Autodesk Inventor part; units mm, degrees
(part 12 of 15)
  arc A5313 (9.6668, 53.008) -> (9.5652, 53.008) centre (9.616, 53.008) ccw
  line L2483 (9.616, 52.992) -> (7.584, 52.992)
  arc A5314 (7.584, 53.0428) -> (7.584, 52.9412) centre (7.584, 52.992) ccw
  arc A5315 (9.616, 52.9412) -> (9.616, 53.0428) centre (9.616, 52.992) ccw
  line L2484 (7.584, 52.992) -> (7.584, 54.008)
  arc A5316 (7.6348, 54.008) -> (7.5332, 54.008) centre (7.584, 54.008) ccw
  arc A5317 (7.5332, 52.992) -> (7.6348, 52.992) centre (7.584, 52.992) ccw
  line L2485 (7.584, 54.008) -> (9.616, 54.008)
  arc A5318 (9.616, 53.9572) -> (9.616, 54.0588) centre (9.616, 54.008) ccw
  arc A5319 (7.584, 54.0588) -> (7.584, 53.9572) centre (7.584, 54.008) ccw
  line L2486 (9.616, 54.008) -> (9.616, 52.992)
  arc A5320 (9.5652, 52.992) -> (9.6668, 52.992) centre (9.616, 52.992) ccw
  arc A5321 (9.6668, 54.008) -> (9.5652, 54.008) centre (9.616, 54.008) ccw
  line L2487 (9.616, 53.992) -> (7.584, 53.992)
  arc A5322 (7.584, 54.0428) -> (7.584, 53.9412) centre (7.584, 53.992) ccw
  arc A5323 (9.616, 53.9412) -> (9.616, 54.0428) centre (9.616, 53.992) ccw
  line L2488 (7.584, 53.992) -> (7.584, 55.008)
  arc A5324 (7.6348, 55.008) -> (7.5332, 55.008) centre (7.584, 55.008) ccw
  arc A5325 (7.5332, 53.992) -> (7.6348, 53.992) centre (7.584, 53.992) ccw
  line L2489 (7.584, 55.008) -> (9.616, 55.008)
  arc A5326 (9.616, 54.9572) -> (9.616, 55.0588) centre (9.616, 55.008) ccw
  arc A5327 (7.584, 55.0588) -> (7.584, 54.9572) centre (7.584, 55.008) ccw
  line L2490 (9.616, 55.008) -> (9.616, 53.992)
  arc A5328 (9.5652, 53.992) -> (9.6668, 53.992) centre (9.616, 53.992) ccw
  arc A5329 (9.6668, 55.008) -> (9.5652, 55.008) centre (9.616, 55.008) ccw
  line L2491 (-9.484, 38.892) -> (-11.516, 38.892)
  arc A5330 (-11.516, 38.9428) -> (-11.516, 38.8412) centre (-11.516, 38.892) ccw
  arc A5331 (-9.484, 38.8412) -> (-9.484, 38.9428) centre (-9.484, 38.892) ccw
  line L2492 (-11.516, 38.892) -> (-11.516, 39.908)
  arc A5332 (-11.4652, 39.908) -> (-11.5668, 39.908) centre (-11.516, 39.908) ccw
  arc A5333 (-11.5668, 38.892) -> (-11.4652, 38.892) centre (-11.516, 38.892) ccw
  line L2493 (-11.516, 39.908) -> (-9.484, 39.908)
  arc A5334 (-9.484, 39.8572) -> (-9.484, 39.9588) centre (-9.484, 39.908) ccw
  arc A5335 (-11.516, 39.9588) -> (-11.516, 39.8572) centre (-11.516, 39.908) ccw
  line L2494 (-9.484, 39.908) -> (-9.484, 38.892)
  arc A5336 (-9.5348, 38.892) -> (-9.4332, 38.892) centre (-9.484, 38.892) ccw
  arc A5337 (-9.4332, 39.908) -> (-9.5348, 39.908) centre (-9.484, 39.908) ccw
  line L2495 (-9.484, 39.892) -> (-11.516, 39.892)
  arc A5338 (-11.516, 39.9428) -> (-11.516, 39.8412) centre (-11.516, 39.892) ccw
  arc A5339 (-9.484, 39.8412) -> (-9.484, 39.9428) centre (-9.484, 39.892) ccw
  line L2496 (-11.516, 39.892) -> (-11.516, 40.908)
  arc A5340 (-11.4652, 40.908) -> (-11.5668, 40.908) centre (-11.516, 40.908) ccw
  arc A5341 (-11.5668, 39.892) -> (-11.4652, 39.892) centre (-11.516, 39.892) ccw
  line L2497 (-11.516, 40.908) -> (-9.484, 40.908)
  arc A5342 (-9.484, 40.8572) -> (-9.484, 40.9588) centre (-9.484, 40.908) ccw
  arc A5343 (-11.516, 40.9588) -> (-11.516, 40.8572) centre (-11.516, 40.908) ccw
  line L2498 (-9.484, 40.908) -> (-9.484, 39.892)
  arc A5344 (-9.5348, 39.892) -> (-9.4332, 39.892) centre (-9.484, 39.892) ccw
  arc A5345 (-9.4332, 40.908) -> (-9.5348, 40.908) centre (-9.484, 40.908) ccw
  line L2499 (11.616, 49.992) -> (9.584, 49.992)
  arc A5346 (9.584, 50.0428) -> (9.584, 49.9412) centre (9.584, 49.992) ccw
  arc A5347 (11.616, 49.9412) -> (11.616, 50.0428) centre (11.616, 49.992) ccw
  line L2500 (9.584, 49.992) -> (9.584, 51.008)
  arc A5348 (9.6348, 51.008) -> (9.5332, 51.008) centre (9.584, 51.008) ccw
  arc A5349 (9.5332, 49.992) -> (9.6348, 49.992) centre (9.584, 49.992) ccw
  line L2501 (9.584, 51.008) -> (11.616, 51.008)
  arc A5350 (11.616, 50.9572) -> (11.616, 51.0588) centre (11.616, 51.008) ccw
  arc A5351 (9.584, 51.0588) -> (9.584, 50.9572) centre (9.584, 51.008) ccw
  line L2502 (11.616, 51.008) -> (11.616, 49.992)
  arc A5352 (11.5652, 49.992) -> (11.6668, 49.992) centre (11.616, 49.992) ccw
  arc A5353 (11.6668, 51.008) -> (11.5652, 51.008) centre (11.616, 51.008) ccw
  line L2503 (11.616, 48.992) -> (9.584, 48.992)
  arc A5354 (9.584, 49.0428) -> (9.584, 48.9412) centre (9.584, 48.992) ccw
  arc A5355 (11.616, 48.9412) -> (11.616, 49.0428) centre (11.616, 48.992) ccw
  line L2504 (9.584, 48.992) -> (9.584, 50.008)
  arc A5356 (9.6348, 50.008) -> (9.5332, 50.008) centre (9.584, 50.008) ccw
  arc A5357 (9.5332, 48.992) -> (9.6348, 48.992) centre (9.584, 48.992) ccw
  line L2505 (9.584, 50.008) -> (11.616, 50.008)
  arc A5358 (11.616, 49.9572) -> (11.616, 50.0588) centre (11.616, 50.008) ccw
  arc A5359 (9.584, 50.0588) -> (9.584, 49.9572) centre (9.584, 50.008) ccw
  line L2506 (11.616, 50.008) -> (11.616, 48.992)
  arc A5360 (11.5652, 48.992) -> (11.6668, 48.992) centre (11.616, 48.992) ccw
  arc A5361 (11.6668, 50.008) -> (11.5652, 50.008) centre (11.616, 50.008) ccw
  line L2507 (11.616, 47.992) -> (9.584, 47.992)
  arc A5362 (9.584, 48.0428) -> (9.584, 47.9412) centre (9.584, 47.992) ccw
  arc A5363 (11.616, 47.9412) -> (11.616, 48.0428) centre (11.616, 47.992) ccw
  line L2508 (9.584, 47.992) -> (9.584, 49.008)
  arc A5364 (9.6348, 49.008) -> (9.5332, 49.008) centre (9.584, 49.008) ccw
  arc A5365 (9.5332, 47.992) -> (9.6348, 47.992) centre (9.584, 47.992) ccw
  line L2509 (9.584, 49.008) -> (11.616, 49.008)
  arc A5366 (11.616, 48.9572) -> (11.616, 49.0588) centre (11.616, 49.008) ccw
  arc A5367 (9.584, 49.0588) -> (9.584, 48.9572) centre (9.584, 49.008) ccw
  line L2510 (11.616, 49.008) -> (11.616, 47.992)
  arc A5368 (11.5652, 47.992) -> (11.6668, 47.992) centre (11.616, 47.992) ccw
  arc A5369 (11.6668, 49.008) -> (11.5652, 49.008) centre (11.616, 49.008) ccw
  line L2511 (9.616, 49.992) -> (7.584, 49.992)
  arc A5370 (7.584, 50.0428) -> (7.584, 49.9412) centre (7.584, 49.992) ccw
  arc A5371 (9.616, 49.9412) -> (9.616, 50.0428) centre (9.616, 49.992) ccw
  line L2512 (7.584, 49.992) -> (7.584, 51.008)
  arc A5372 (7.6348, 51.008) -> (7.5332, 51.008) centre (7.584, 51.008) ccw
  arc A5373 (7.5332, 49.992) -> (7.6348, 49.992) centre (7.584, 49.992) ccw
  line L2513 (7.584, 51.008) -> (9.616, 51.008)
  arc A5374 (9.616, 50.9572) -> (9.616, 51.0588) centre (9.616, 51.008) ccw
  arc A5375 (7.584, 51.0588) -> (7.584, 50.9572) centre (7.584, 51.008) ccw
  line L2514 (9.616, 51.008) -> (9.616, 49.992)
  arc A5376 (9.5652, 49.992) -> (9.6668, 49.992) centre (9.616, 49.992) ccw
  arc A5377 (9.6668, 51.008) -> (9.5652, 51.008) centre (9.616, 51.008) ccw
  line L2515 (63.534, 34.908) -> (65.566, 34.908)
  arc A5378 (65.566, 34.8572) -> (65.566, 34.9588) centre (65.566, 34.908) ccw
  arc A5379 (63.534, 34.9588) -> (63.534, 34.8572) centre (63.534, 34.908) ccw
  line L2516 (65.566, 34.908) -> (65.566, 33.892)
  arc A5380 (65.5152, 33.892) -> (65.6168, 33.892) centre (65.566, 33.892) ccw
  arc A5381 (65.6168, 34.908) -> (65.5152, 34.908) centre (65.566, 34.908) ccw
  line L2517 (65.566, 33.892) -> (63.534, 33.892)
  arc A5382 (63.534, 33.9428) -> (63.534, 33.8412) centre (63.534, 33.892) ccw
  arc A5383 (65.566, 33.8412) -> (65.566, 33.9428) centre (65.566, 33.892) ccw
  line L2518 (63.534, 33.892) -> (63.534, 34.908)
  arc A5384 (63.5848, 34.908) -> (63.4832, 34.908) centre (63.534, 34.908) ccw
  arc A5385 (63.4832, 33.892) -> (63.5848, 33.892) centre (63.534, 33.892) ccw
  line L2519 (65.566, 34.892) -> (63.534, 34.892)
  arc A5386 (63.534, 34.9428) -> (63.534, 34.8412) centre (63.534, 34.892) ccw
  arc A5387 (65.566, 34.8412) -> (65.566, 34.9428) centre (65.566, 34.892) ccw
  line L2520 (63.534, 34.892) -> (63.534, 35.908)
  arc A5388 (63.5848, 35.908) -> (63.4832, 35.908) centre (63.534, 35.908) ccw
  arc A5389 (63.4832, 34.892) -> (63.5848, 34.892) centre (63.534, 34.892) ccw
  line L2521 (63.534, 35.908) -> (65.566, 35.908)
  arc A5390 (65.566, 35.8572) -> (65.566, 35.9588) centre (65.566, 35.908) ccw
  arc A5391 (63.534, 35.9588) -> (63.534, 35.8572) centre (63.534, 35.908) ccw
  line L2522 (65.566, 35.908) -> (65.566, 34.892)
  arc A5392 (65.5152, 34.892) -> (65.6168, 34.892) centre (65.566, 34.892) ccw
  arc A5393 (65.6168, 35.908) -> (65.5152, 35.908) centre (65.566, 35.908) ccw
  line L2523 (63.334, 56.308) -> (65.366, 56.308)
  arc A5394 (65.366, 56.2572) -> (65.366, 56.3588) centre (65.366, 56.308) ccw
  arc A5395 (63.334, 56.3588) -> (63.334, 56.2572) centre (63.334, 56.308) ccw
  line L2524 (65.366, 56.308) -> (65.366, 55.292)
  arc A5396 (65.3152, 55.292) -> (65.4168, 55.292) centre (65.366, 55.292) ccw
  arc A5397 (65.4168, 56.308) -> (65.3152, 56.308) centre (65.366, 56.308) ccw
  line L2525 (65.366, 55.292) -> (63.334, 55.292)
  arc A5398 (63.334, 55.3428) -> (63.334, 55.2412) centre (63.334, 55.292) ccw
  arc A5399 (65.366, 55.2412) -> (65.366, 55.3428) centre (65.366, 55.292) ccw
  line L2526 (63.334, 55.292) -> (63.334, 56.308)
  arc A5400 (63.3848, 56.308) -> (63.2832, 56.308) centre (63.334, 56.308) ccw
  arc A5401 (63.2832, 55.292) -> (63.3848, 55.292) centre (63.334, 55.292) ccw
  line L2527 (9.584, 47.008) -> (11.616, 47.008)
  arc A5402 (11.616, 46.9572) -> (11.616, 47.0588) centre (11.616, 47.008) ccw
  arc A5403 (9.584, 47.0588) -> (9.584, 46.9572) centre (9.584, 47.008) ccw
  line L2528 (11.616, 47.008) -> (11.616, 45.992)
  arc A5404 (11.5652, 45.992) -> (11.6668, 45.992) centre (11.616, 45.992) ccw
  arc A5405 (11.6668, 47.008) -> (11.5652, 47.008) centre (11.616, 47.008) ccw
  line L2529 (11.616, 45.992) -> (9.584, 45.992)
  arc A5406 (9.584, 46.0428) -> (9.584, 45.9412) centre (9.584, 45.992) ccw
  arc A5407 (11.616, 45.9412) -> (11.616, 46.0428) centre (11.616, 45.992) ccw
  line L2530 (9.584, 45.992) -> (9.584, 47.008)
  arc A5408 (9.6348, 47.008) -> (9.5332, 47.008) centre (9.584, 47.008) ccw
  arc A5409 (9.5332, 45.992) -> (9.6348, 45.992) centre (9.584, 45.992) ccw
  line L2531 (11.616, 46.992) -> (9.584, 46.992)
  arc A5410 (9.584, 47.0428) -> (9.584, 46.9412) centre (9.584, 46.992) ccw
  arc A5411 (11.616, 46.9412) -> (11.616, 47.0428) centre (11.616, 46.992) ccw
  line L2532 (9.584, 46.992) -> (9.584, 48.008)
  arc A5412 (9.6348, 48.008) -> (9.5332, 48.008) centre (9.584, 48.008) ccw
  arc A5413 (9.5332, 46.992) -> (9.6348, 46.992) centre (9.584, 46.992) ccw
  line L2533 (9.584, 48.008) -> (11.616, 48.008)
  arc A5414 (11.616, 47.9572) -> (11.616, 48.0588) centre (11.616, 48.008) ccw
  arc A5415 (9.584, 48.0588) -> (9.584, 47.9572) centre (9.584, 48.008) ccw
  line L2534 (11.616, 48.008) -> (11.616, 46.992)
  arc A5416 (11.5652, 46.992) -> (11.6668, 46.992) centre (11.616, 46.992) ccw
  arc A5417 (11.6668, 48.008) -> (11.5652, 48.008) centre (11.616, 48.008) ccw
  line L2535 (-2.616, 55.708) -> (-0.584, 55.708)
  arc A5418 (-0.584, 55.6572) -> (-0.584, 55.7588) centre (-0.584, 55.708) ccw
  arc A5419 (-2.616, 55.7588) -> (-2.616, 55.6572) centre (-2.616, 55.708) ccw
  line L2536 (-0.584, 55.708) -> (-0.584, 54.692)
  arc A5420 (-0.6348, 54.692) -> (-0.5332, 54.692) centre (-0.584, 54.692) ccw
  arc A5421 (-0.5332, 55.708) -> (-0.6348, 55.708) centre (-0.584, 55.708) ccw
  line L2537 (-0.584, 54.692) -> (-2.616, 54.692)
  arc A5422 (-2.616, 54.7428) -> (-2.616, 54.6412) centre (-2.616, 54.692) ccw
  arc A5423 (-0.584, 54.6412) -> (-0.584, 54.7428) centre (-0.584, 54.692) ccw
  line L2538 (-2.616, 54.692) -> (-2.616, 55.708)
  arc A5424 (-2.5652, 55.708) -> (-2.6668, 55.708) centre (-2.616, 55.708) ccw
  arc A5425 (-2.6668, 54.692) -> (-2.5652, 54.692) centre (-2.616, 54.692) ccw
  line L2539 (4.508, 37.216) -> (4.508, 35.184)
  arc A5426 (4.4572, 35.184) -> (4.5588, 35.184) centre (4.508, 35.184) ccw
  arc A5427 (4.5588, 37.216) -> (4.4572, 37.216) centre (4.508, 37.216) ccw
  line L2540 (4.508, 35.184) -> (3.492, 35.184)
  arc A5428 (3.492, 35.2348) -> (3.492, 35.1332) centre (3.492, 35.184) ccw
  arc A5429 (4.508, 35.1332) -> (4.508, 35.2348) centre (4.508, 35.184) ccw
  line L2541 (3.492, 35.184) -> (3.492, 37.216)
  arc A5430 (3.5428, 37.216) -> (3.4412, 37.216) centre (3.492, 37.216) ccw
  arc A5431 (3.4412, 35.184) -> (3.5428, 35.184) centre (3.492, 35.184) ccw
  line L2542 (3.492, 37.216) -> (4.508, 37.216)
  arc A5432 (4.508, 37.1652) -> (4.508, 37.2668) centre (4.508, 37.216) ccw
  arc A5433 (3.492, 37.2668) -> (3.492, 37.1652) centre (3.492, 37.216) ccw
  line L2543 (3.308, 37.216) -> (3.308, 35.184)
  arc A5434 (3.2572, 35.184) -> (3.3588, 35.184) centre (3.308, 35.184) ccw
  arc A5435 (3.3588, 37.216) -> (3.2572, 37.216) centre (3.308, 37.216) ccw
  line L2544 (3.308, 35.184) -> (2.292, 35.184)
  arc A5436 (2.292, 35.2348) -> (2.292, 35.1332) centre (2.292, 35.184) ccw
  arc A5437 (3.308, 35.1332) -> (3.308, 35.2348) centre (3.308, 35.184) ccw
  line L2545 (2.292, 35.184) -> (2.292, 37.216)
  arc A5438 (2.3428, 37.216) -> (2.2412, 37.216) centre (2.292, 37.216) ccw
  arc A5439 (2.2412, 35.184) -> (2.3428, 35.184) centre (2.292, 35.184) ccw
  line L2546 (2.292, 37.216) -> (3.308, 37.216)
  arc A5440 (3.308, 37.1652) -> (3.308, 37.2668) centre (3.308, 37.216) ccw
  arc A5441 (2.292, 37.2668) -> (2.292, 37.1652) centre (2.292, 37.216) ccw
  line L2547 (1.292, 37.784) -> (1.292, 39.816)
  arc A5442 (1.3428, 39.816) -> (1.2412, 39.816) centre (1.292, 39.816) ccw
  arc A5443 (1.2412, 37.784) -> (1.3428, 37.784) centre (1.292, 37.784) ccw
  line L2548 (1.292, 39.816) -> (2.308, 39.816)
  arc A5444 (2.308, 39.7652) -> (2.308, 39.8668) centre (2.308, 39.816) ccw
  arc A5445 (1.292, 39.8668) -> (1.292, 39.7652) centre (1.292, 39.816) ccw
  line L2549 (2.308, 39.816) -> (2.308, 37.784)
  arc A5446 (2.2572, 37.784) -> (2.3588, 37.784) centre (2.308, 37.784) ccw
  arc A5447 (2.3588, 39.816) -> (2.2572, 39.816) centre (2.308, 39.816) ccw
  line L2550 (2.308, 37.784) -> (1.292, 37.784)
  arc A5448 (1.292, 37.8348) -> (1.292, 37.7332) centre (1.292, 37.784) ccw
  arc A5449 (2.308, 37.7332) -> (2.308, 37.8348) centre (2.308, 37.784) ccw
  line L2551 (61.234, 56.308) -> (63.266, 56.308)
  arc A5450 (63.266, 56.2572) -> (63.266, 56.3588) centre (63.266, 56.308) ccw
  arc A5451 (61.234, 56.3588) -> (61.234, 56.2572) centre (61.234, 56.308) ccw
  line L2552 (63.266, 56.308) -> (63.266, 55.292)
  arc A5452 (63.2152, 55.292) -> (63.3168, 55.292) centre (63.266, 55.292) ccw
  arc A5453 (63.3168, 56.308) -> (63.2152, 56.308) centre (63.266, 56.308) ccw
  line L2553 (63.266, 55.292) -> (61.234, 55.292)
  arc A5454 (61.234, 55.3428) -> (61.234, 55.2412) centre (61.234, 55.292) ccw
  arc A5455 (63.266, 55.2412) -> (63.266, 55.3428) centre (63.266, 55.292) ccw
  line L2554 (61.234, 55.292) -> (61.234, 56.308)
  arc A5456 (61.2848, 56.308) -> (61.1832, 56.308) centre (61.234, 56.308) ccw
  arc A5457 (61.1832, 55.292) -> (61.2848, 55.292) centre (61.234, 55.292) ccw
  line L2555 (67.466, 55.292) -> (65.434, 55.292)
  arc A5458 (65.434, 55.3428) -> (65.434, 55.2412) centre (65.434, 55.292) ccw
  arc A5459 (67.466, 55.2412) -> (67.466, 55.3428) centre (67.466, 55.292) ccw
  line L2556 (65.434, 55.292) -> (65.434, 56.308)
  arc A5460 (65.4848, 56.308) -> (65.3832, 56.308) centre (65.434, 56.308) ccw
  arc A5461 (65.3832, 55.292) -> (65.4848, 55.292) centre (65.434, 55.292) ccw
  line L2557 (65.434, 56.308) -> (67.466, 56.308)
  arc A5462 (67.466, 56.2572) -> (67.466, 56.3588) centre (67.466, 56.308) ccw
  arc A5463 (65.434, 56.3588) -> (65.434, 56.2572) centre (65.434, 56.308) ccw
  line L2558 (67.466, 56.308) -> (67.466, 55.292)
  arc A5464 (67.4152, 55.292) -> (67.5168, 55.292) centre (67.466, 55.292) ccw
  arc A5465 (67.5168, 56.308) -> (67.4152, 56.308) centre (67.466, 56.308) ccw
  line L2559 (23.616, -96.808) -> (21.584, -96.808)
  arc A5466 (21.584, -96.7572) -> (21.584, -96.8588) centre (21.584, -96.808) ccw
  arc A5467 (23.616, -96.8588) -> (23.616, -96.7572) centre (23.616, -96.808) ccw
  line L2560 (21.584, -96.808) -> (21.584, -95.792)
  arc A5468 (21.6348, -95.792) -> (21.5332, -95.792) centre (21.584, -95.792) ccw
  arc A5469 (21.5332, -96.808) -> (21.6348, -96.808) centre (21.584, -96.808) ccw
  line L2561 (21.584, -95.792) -> (23.616, -95.792)
  arc A5470 (23.616, -95.8428) -> (23.616, -95.7412) centre (23.616, -95.792) ccw
  arc A5471 (21.584, -95.7412) -> (21.584, -95.8428) centre (21.584, -95.792) ccw
  line L2562 (23.616, -95.792) -> (23.616, -96.808)
  arc A5472 (23.5652, -96.808) -> (23.6668, -96.808) centre (23.616, -96.808) ccw
  arc A5473 (23.6668, -95.792) -> (23.5652, -95.792) centre (23.616, -95.792) ccw
  line L2563 (16.308, -84.484) -> (16.308, -86.516)
  arc A5474 (16.2572, -86.516) -> (16.3588, -86.516) centre (16.308, -86.516) ccw
  arc A5475 (16.3588, -84.484) -> (16.2572, -84.484) centre (16.308, -84.484) ccw
  line L2564 (16.308, -86.516) -> (15.292, -86.516)
  arc A5476 (15.292, -86.4652) -> (15.292, -86.5668) centre (15.292, -86.516) ccw
  arc A5477 (16.308, -86.5668) -> (16.308, -86.4652) centre (16.308, -86.516) ccw
  line L2565 (15.292, -86.516) -> (15.292, -84.484)
  arc A5478 (15.3428, -84.484) -> (15.2412, -84.484) centre (15.292, -84.484) ccw
  arc A5479 (15.2412, -86.516) -> (15.3428, -86.516) centre (15.292, -86.516) ccw
  line L2566 (15.292, -84.484) -> (16.308, -84.484)
  arc A5480 (16.308, -84.5348) -> (16.308, -84.4332) centre (16.308, -84.484) ccw
  arc A5481 (15.292, -84.4332) -> (15.292, -84.5348) centre (15.292, -84.484) ccw
  line L2567 (23.792, -96.816) -> (23.792, -94.784)
  arc A5482 (23.8428, -94.784) -> (23.7412, -94.784) centre (23.792, -94.784) ccw
  arc A5483 (23.7412, -96.816) -> (23.8428, -96.816) centre (23.792, -96.816) ccw
  line L2568 (23.792, -94.784) -> (24.808, -94.784)
  arc A5484 (24.808, -94.8348) -> (24.808, -94.7332) centre (24.808, -94.784) ccw
  arc A5485 (23.792, -94.7332) -> (23.792, -94.8348) centre (23.792, -94.784) ccw
  line L2569 (24.808, -94.784) -> (24.808, -96.816)
  arc A5486 (24.7572, -96.816) -> (24.8588, -96.816) centre (24.808, -96.816) ccw
  arc A5487 (24.8588, -94.784) -> (24.7572, -94.784) centre (24.808, -94.784) ccw
  line L2570 (24.808, -96.816) -> (23.792, -96.816)
  arc A5488 (23.792, -96.7652) -> (23.792, -96.8668) centre (23.792, -96.816) ccw
  arc A5489 (24.808, -96.8668) -> (24.808, -96.7652) centre (24.808, -96.816) ccw
  line L2571 (23.616, -93.708) -> (21.584, -93.708)
  arc A5490 (21.584, -93.6572) -> (21.584, -93.7588) centre (21.584, -93.708) ccw
  arc A5491 (23.616, -93.7588) -> (23.616, -93.6572) centre (23.616, -93.708) ccw
  line L2572 (21.584, -93.708) -> (21.584, -92.692)
  arc A5492 (21.6348, -92.692) -> (21.5332, -92.692) centre (21.584, -92.692) ccw
  arc A5493 (21.5332, -93.708) -> (21.6348, -93.708) centre (21.584, -93.708) ccw
  line L2573 (21.584, -92.692) -> (23.616, -92.692)
  arc A5494 (23.616, -92.7428) -> (23.616, -92.6412) centre (23.616, -92.692) ccw
  arc A5495 (21.584, -92.6412) -> (21.584, -92.7428) centre (21.584, -92.692) ccw
  line L2574 (23.616, -92.692) -> (23.616, -93.708)
  arc A5496 (23.5652, -93.708) -> (23.6668, -93.708) centre (23.616, -93.708) ccw
  arc A5497 (23.6668, -92.692) -> (23.5652, -92.692) centre (23.616, -92.692) ccw
  line L2575 (23.792, -93.716) -> (23.792, -91.684)
  arc A5498 (23.8428, -91.684) -> (23.7412, -91.684) centre (23.792, -91.684) ccw
  arc A5499 (23.7412, -93.716) -> (23.8428, -93.716) centre (23.792, -93.716) ccw
  line L2576 (23.792, -91.684) -> (24.808, -91.684)
  arc A5500 (24.808, -91.7348) -> (24.808, -91.6332) centre (24.808, -91.684) ccw
  arc A5501 (23.792, -91.6332) -> (23.792, -91.7348) centre (23.792, -91.684) ccw
  line L2577 (24.808, -91.684) -> (24.808, -93.716)
  arc A5502 (24.7572, -93.716) -> (24.8588, -93.716) centre (24.808, -93.716) ccw
  arc A5503 (24.8588, -91.684) -> (24.7572, -91.684) centre (24.808, -91.684) ccw
  line L2578 (24.808, -93.716) -> (23.792, -93.716)
  arc A5504 (23.792, -93.6652) -> (23.792, -93.7668) centre (23.792, -93.716) ccw
  arc A5505 (24.808, -93.7668) -> (24.808, -93.6652) centre (24.808, -93.716) ccw
  line L2579 (-7.216, -13.092) -> (-5.184, -13.092)
  arc A5506 (-5.184, -13.1428) -> (-5.184, -13.0412) centre (-5.184, -13.092) ccw
  arc A5507 (-7.216, -13.0412) -> (-7.216, -13.1428) centre (-7.216, -13.092) ccw
  line L2580 (-5.184, -13.092) -> (-5.184, -14.108)
  arc A5508 (-5.2348, -14.108) -> (-5.1332, -14.108) centre (-5.184, -14.108) ccw
  arc A5509 (-5.1332, -13.092) -> (-5.2348, -13.092) centre (-5.184, -13.092) ccw
  line L2581 (-5.184, -14.108) -> (-7.216, -14.108)
  arc A5510 (-7.216, -14.0572) -> (-7.216, -14.1588) centre (-7.216, -14.108) ccw
  arc A5511 (-5.184, -14.1588) -> (-5.184, -14.0572) centre (-5.184, -14.108) ccw
  line L2582 (-7.216, -14.108) -> (-7.216, -13.092)
  arc A5512 (-7.1652, -13.092) -> (-7.2668, -13.092) centre (-7.216, -13.092) ccw
  arc A5513 (-7.2668, -14.108) -> (-7.1652, -14.108) centre (-7.216, -14.108) ccw
  line L2583 (-7.216, -14.092) -> (-5.184, -14.092)
  arc A5514 (-5.184, -14.1428) -> (-5.184, -14.0412) centre (-5.184, -14.092) ccw
  arc A5515 (-7.216, -14.0412) -> (-7.216, -14.1428) centre (-7.216, -14.092) ccw
  line L2584 (-5.184, -14.092) -> (-5.184, -15.108)
  arc A5516 (-5.2348, -15.108) -> (-5.1332, -15.108) centre (-5.184, -15.108) ccw
  arc A5517 (-5.1332, -14.092) -> (-5.2348, -14.092) centre (-5.184, -14.092) ccw
  line L2585 (-5.184, -15.108) -> (-7.216, -15.108)
  arc A5518 (-7.216, -15.0572) -> (-7.216, -15.1588) centre (-7.216, -15.108) ccw
  arc A5519 (-5.184, -15.1588) -> (-5.184, -15.0572) centre (-5.184, -15.108) ccw
  line L2586 (-7.216, -15.108) -> (-7.216, -14.092)
  arc A5520 (-7.1652, -14.092) -> (-7.2668, -14.092) centre (-7.216, -14.092) ccw
  arc A5521 (-7.2668, -15.108) -> (-7.1652, -15.108) centre (-7.216, -15.108) ccw
  line L2587 (-1.784, -19.108) -> (-3.816, -19.108)
  arc A5522 (-3.816, -19.0572) -> (-3.816, -19.1588) centre (-3.816, -19.108) ccw
  arc A5523 (-1.784, -19.1588) -> (-1.784, -19.0572) centre (-1.784, -19.108) ccw
  line L2588 (-3.816, -19.108) -> (-3.816, -18.092)
  arc A5524 (-3.7652, -18.092) -> (-3.8668, -18.092) centre (-3.816, -18.092) ccw
  arc A5525 (-3.8668, -19.108) -> (-3.7652, -19.108) centre (-3.816, -19.108) ccw
  line L2589 (-3.816, -18.092) -> (-1.784, -18.092)
  arc A5526 (-1.784, -18.1428) -> (-1.784, -18.0412) centre (-1.784, -18.092) ccw
  arc A5527 (-3.816, -18.0412) -> (-3.816, -18.1428) centre (-3.816, -18.092) ccw
  line L2590 (-1.784, -18.092) -> (-1.784, -19.108)
  arc A5528 (-1.8348, -19.108) -> (-1.7332, -19.108) centre (-1.784, -19.108) ccw
  arc A5529 (-1.7332, -18.092) -> (-1.8348, -18.092) centre (-1.784, -18.092) ccw
  line L2591 (-7.216, -18.092) -> (-5.184, -18.092)
  arc A5530 (-5.184, -18.1428) -> (-5.184, -18.0412) centre (-5.184, -18.092) ccw
  arc A5531 (-7.216, -18.0412) -> (-7.216, -18.1428) centre (-7.216, -18.092) ccw
  line L2592 (-5.184, -18.092) -> (-5.184, -19.108)
  arc A5532 (-5.2348, -19.108) -> (-5.1332, -19.108) centre (-5.184, -19.108) ccw
  arc A5533 (-5.1332, -18.092) -> (-5.2348, -18.092) centre (-5.184, -18.092) ccw
  line L2593 (-5.184, -19.108) -> (-7.216, -19.108)
  arc A5534 (-7.216, -19.0572) -> (-7.216, -19.1588) centre (-7.216, -19.108) ccw
  arc A5535 (-5.184, -19.1588) -> (-5.184, -19.0572) centre (-5.184, -19.108) ccw
  line L2594 (-7.216, -19.108) -> (-7.216, -18.092)
  arc A5536 (-7.1652, -18.092) -> (-7.2668, -18.092) centre (-7.216, -18.092) ccw
  arc A5537 (-7.2668, -19.108) -> (-7.1652, -19.108) centre (-7.216, -19.108) ccw
  line L2595 (-1.784, -15.108) -> (-3.816, -15.108)
  arc A5538 (-3.816, -15.0572) -> (-3.816, -15.1588) centre (-3.816, -15.108) ccw
  arc A5539 (-1.784, -15.1588) -> (-1.784, -15.0572) centre (-1.784, -15.108) ccw
  line L2596 (-3.816, -15.108) -> (-3.816, -14.092)
  arc A5540 (-3.7652, -14.092) -> (-3.8668, -14.092) centre (-3.816, -14.092) ccw
  arc A5541 (-3.8668, -15.108) -> (-3.7652, -15.108) centre (-3.816, -15.108) ccw
  line L2597 (-3.816, -14.092) -> (-1.784, -14.092)
  arc A5542 (-1.784, -14.1428) -> (-1.784, -14.0412) centre (-1.784, -14.092) ccw
  arc A5543 (-3.816, -14.0412) -> (-3.816, -14.1428) centre (-3.816, -14.092) ccw
  line L2598 (-1.784, -14.092) -> (-1.784, -15.108)
  arc A5544 (-1.8348, -15.108) -> (-1.7332, -15.108) centre (-1.784, -15.108) ccw
  arc A5545 (-1.7332, -14.092) -> (-1.8348, -14.092) centre (-1.784, -14.092) ccw
  line L2599 (-7.216, -22.092) -> (-5.184, -22.092)
  arc A5546 (-5.184, -22.1428) -> (-5.184, -22.0412) centre (-5.184, -22.092) ccw
  arc A5547 (-7.216, -22.0412) -> (-7.216, -22.1428) centre (-7.216, -22.092) ccw
  line L2600 (-5.184, -22.092) -> (-5.184, -23.108)
  arc A5548 (-5.2348, -23.108) -> (-5.1332, -23.108) centre (-5.184, -23.108) ccw
  arc A5549 (-5.1332, -22.092) -> (-5.2348, -22.092) centre (-5.184, -22.092) ccw
  line L2601 (-5.184, -23.108) -> (-7.216, -23.108)
  arc A5550 (-7.216, -23.0572) -> (-7.216, -23.1588) centre (-7.216, -23.108) ccw
  arc A5551 (-5.184, -23.1588) -> (-5.184, -23.0572) centre (-5.184, -23.108) ccw
  line L2602 (-7.216, -23.108) -> (-7.216, -22.092)
  arc A5552 (-7.1652, -22.092) -> (-7.2668, -22.092) centre (-7.216, -22.092) ccw
  arc A5553 (-7.2668, -23.108) -> (-7.1652, -23.108) centre (-7.216, -23.108) ccw
  line L2603 (-7.216, -24.092) -> (-5.184, -24.092)
  arc A5554 (-5.184, -24.1428) -> (-5.184, -24.0412) centre (-5.184, -24.092) ccw
  arc A5555 (-7.216, -24.0412) -> (-7.216, -24.1428) centre (-7.216, -24.092) ccw
  line L2604 (-5.184, -24.092) -> (-5.184, -25.108)
  arc A5556 (-5.2348, -25.108) -> (-5.1332, -25.108) centre (-5.184, -25.108) ccw
  arc A5557 (-5.1332, -24.092) -> (-5.2348, -24.092) centre (-5.184, -24.092) ccw
  line L2605 (-5.184, -25.108) -> (-7.216, -25.108)
  arc A5558 (-7.216, -25.0572) -> (-7.216, -25.1588) centre (-7.216, -25.108) ccw
  arc A5559 (-5.184, -25.1588) -> (-5.184, -25.0572) centre (-5.184, -25.108) ccw
  line L2606 (-7.216, -25.108) -> (-7.216, -24.092)
  arc A5560 (-7.1652, -24.092) -> (-7.2668, -24.092) centre (-7.216, -24.092) ccw
  arc A5561 (-7.2668, -25.108) -> (-7.1652, -25.108) centre (-7.216, -25.108) ccw
  line L2607 (-7.216, -19.092) -> (-5.184, -19.092)
  arc A5562 (-5.184, -19.1428) -> (-5.184, -19.0412) centre (-5.184, -19.092) ccw
  arc A5563 (-7.216, -19.0412) -> (-7.216, -19.1428) centre (-7.216, -19.092) ccw
  line L2608 (-5.184, -19.092) -> (-5.184, -20.108)
  arc A5564 (-5.2348, -20.108) -> (-5.1332, -20.108) centre (-5.184, -20.108) ccw
  arc A5565 (-5.1332, -19.092) -> (-5.2348, -19.092) centre (-5.184, -19.092) ccw
  line L2609 (-5.184, -20.108) -> (-7.216, -20.108)
  arc A5566 (-7.216, -20.0572) -> (-7.216, -20.1588) centre (-7.216, -20.108) ccw
  arc A5567 (-5.184, -20.1588) -> (-5.184, -20.0572) centre (-5.184, -20.108) ccw
  line L2610 (-7.216, -20.108) -> (-7.216, -19.092)
  arc A5568 (-7.1652, -19.092) -> (-7.2668, -19.092) centre (-7.216, -19.092) ccw
  arc A5569 (-7.2668, -20.108) -> (-7.1652, -20.108) centre (-7.216, -20.108) ccw
  line L2611 (-7.216, -21.092) -> (-5.184, -21.092)
  arc A5570 (-5.184, -21.1428) -> (-5.184, -21.0412) centre (-5.184, -21.092) ccw
  arc A5571 (-7.216, -21.0412) -> (-7.216, -21.1428) centre (-7.216, -21.092) ccw
  line L2612 (-5.184, -21.092) -> (-5.184, -22.108)
  arc A5572 (-5.2348, -22.108) -> (-5.1332, -22.108) centre (-5.184, -22.108) ccw
  arc A5573 (-5.1332, -21.092) -> (-5.2348, -21.092) centre (-5.184, -21.092) ccw
  line L2613 (-5.184, -22.108) -> (-7.216, -22.108)
  arc A5574 (-7.216, -22.0572) -> (-7.216, -22.1588) centre (-7.216, -22.108) ccw
  arc A5575 (-5.184, -22.1588) -> (-5.184, -22.0572) centre (-5.184, -22.108) ccw
  line L2614 (-7.216, -22.108) -> (-7.216, -21.092)
  arc A5576 (-7.1652, -21.092) -> (-7.2668, -21.092) centre (-7.216, -21.092) ccw
  arc A5577 (-7.2668, -22.108) -> (-7.1652, -22.108) centre (-7.216, -22.108) ccw
  line L2615 (-7.216, -17.092) -> (-5.184, -17.092)
  arc A5578 (-5.184, -17.1428) -> (-5.184, -17.0412) centre (-5.184, -17.092) ccw
  arc A5579 (-7.216, -17.0412) -> (-7.216, -17.1428) centre (-7.216, -17.092) ccw
  line L2616 (-5.184, -17.092) -> (-5.184, -18.108)
  arc A5580 (-5.2348, -18.108) -> (-5.1332, -18.108) centre (-5.184, -18.108) ccw
  arc A5581 (-5.1332, -17.092) -> (-5.2348, -17.092) centre (-5.184, -17.092) ccw
  line L2617 (-5.184, -18.108) -> (-7.216, -18.108)
  arc A5582 (-7.216, -18.0572) -> (-7.216, -18.1588) centre (-7.216, -18.108) ccw
  arc A5583 (-5.184, -18.1588) -> (-5.184, -18.0572) centre (-5.184, -18.108) ccw
  line L2618 (-7.216, -18.108) -> (-7.216, -17.092)
  arc A5584 (-7.1652, -17.092) -> (-7.2668, -17.092) centre (-7.216, -17.092) ccw
  arc A5585 (-7.2668, -18.108) -> (-7.1652, -18.108) centre (-7.216, -18.108) ccw
  line L2619 (-1.784, -17.108) -> (-3.816, -17.108)
  arc A5586 (-3.816, -17.0572) -> (-3.816, -17.1588) centre (-3.816, -17.108) ccw
  arc A5587 (-1.784, -17.1588) -> (-1.784, -17.0572) centre (-1.784, -17.108) ccw
  line L2620 (-3.816, -17.108) -> (-3.816, -16.092)
  arc A5588 (-3.7652, -16.092) -> (-3.8668, -16.092) centre (-3.816, -16.092) ccw
  arc A5589 (-3.8668, -17.108) -> (-3.7652, -17.108) centre (-3.816, -17.108) ccw
  line L2621 (-3.816, -16.092) -> (-1.784, -16.092)
  arc A5590 (-1.784, -16.1428) -> (-1.784, -16.0412) centre (-1.784, -16.092) ccw
  arc A5591 (-3.816, -16.0412) -> (-3.816, -16.1428) centre (-3.816, -16.092) ccw
  line L2622 (-1.784, -16.092) -> (-1.784, -17.108)
  arc A5592 (-1.8348, -17.108) -> (-1.7332, -17.108) centre (-1.784, -17.108) ccw
  arc A5593 (-1.7332, -16.092) -> (-1.8348, -16.092) centre (-1.784, -16.092) ccw
  line L2623 (-7.216, -16.092) -> (-5.184, -16.092)
  arc A5594 (-5.184, -16.1428) -> (-5.184, -16.0412) centre (-5.184, -16.092) ccw
  arc A5595 (-7.216, -16.0412) -> (-7.216, -16.1428) centre (-7.216, -16.092) ccw
  line L2624 (-5.184, -16.092) -> (-5.184, -17.108)
  arc A5596 (-5.2348, -17.108) -> (-5.1332, -17.108) centre (-5.184, -17.108) ccw
  arc A5597 (-5.1332, -16.092) -> (-5.2348, -16.092) centre (-5.184, -16.092) ccw
  line L2625 (-5.184, -17.108) -> (-7.216, -17.108)
  arc A5598 (-7.216, -17.0572) -> (-7.216, -17.1588) centre (-7.216, -17.108) ccw
  arc A5599 (-5.184, -17.1588) -> (-5.184, -17.0572) centre (-5.184, -17.108) ccw
  line L2626 (-7.216, -17.108) -> (-7.216, -16.092)
  arc A5600 (-7.1652, -16.092) -> (-7.2668, -16.092) centre (-7.216, -16.092) ccw
  arc A5601 (-7.2668, -17.108) -> (-7.1652, -17.108) centre (-7.216, -17.108) ccw
  line L2627 (-1.784, -22.108) -> (-3.816, -22.108)
  arc A5602 (-3.816, -22.0572) -> (-3.816, -22.1588) centre (-3.816, -22.108) ccw
  arc A5603 (-1.784, -22.1588) -> (-1.784, -22.0572) centre (-1.784, -22.108) ccw
  line L2628 (-3.816, -22.108) -> (-3.816, -21.092)
  arc A5604 (-3.7652, -21.092) -> (-3.8668, -21.092) centre (-3.816, -21.092) ccw
  arc A5605 (-3.8668, -22.108) -> (-3.7652, -22.108) centre (-3.816, -22.108) ccw
  line L2629 (-3.816, -21.092) -> (-1.784, -21.092)
  arc A5606 (-1.784, -21.1428) -> (-1.784, -21.0412) centre (-1.784, -21.092) ccw
  arc A5607 (-3.816, -21.0412) -> (-3.816, -21.1428) centre (-3.816, -21.092) ccw
  line L2630 (-1.784, -21.092) -> (-1.784, -22.108)
  arc A5608 (-1.8348, -22.108) -> (-1.7332, -22.108) centre (-1.784, -22.108) ccw
  arc A5609 (-1.7332, -21.092) -> (-1.8348, -21.092) centre (-1.784, -21.092) ccw
  line L2631 (-1.784, -16.108) -> (-3.816, -16.108)
  arc A5610 (-3.816, -16.0572) -> (-3.816, -16.1588) centre (-3.816, -16.108) ccw
  arc A5611 (-1.784, -16.1588) -> (-1.784, -16.0572) centre (-1.784, -16.108) ccw
  line L2632 (-3.816, -16.108) -> (-3.816, -15.092)
  arc A5612 (-3.7652, -15.092) -> (-3.8668, -15.092) centre (-3.816, -15.092) ccw
  arc A5613 (-3.8668, -16.108) -> (-3.7652, -16.108) centre (-3.816, -16.108) ccw
  line L2633 (-3.816, -15.092) -> (-1.784, -15.092)
  arc A5614 (-1.784, -15.1428) -> (-1.784, -15.0412) centre (-1.784, -15.092) ccw
  arc A5615 (-3.816, -15.0412) -> (-3.816, -15.1428) centre (-3.816, -15.092) ccw
  line L2634 (-1.784, -15.092) -> (-1.784, -16.108)
  arc A5616 (-1.8348, -16.108) -> (-1.7332, -16.108) centre (-1.784, -16.108) ccw
  arc A5617 (-1.7332, -15.092) -> (-1.8348, -15.092) centre (-1.784, -15.092) ccw
  line L2635 (-1.784, -24.108) -> (-3.816, -24.108)
  arc A5618 (-3.816, -24.0572) -> (-3.816, -24.1588) centre (-3.816, -24.108) ccw
  arc A5619 (-1.784, -24.1588) -> (-1.784, -24.0572) centre (-1.784, -24.108) ccw
  line L2636 (-3.816, -24.108) -> (-3.816, -23.092)
  arc A5620 (-3.7652, -23.092) -> (-3.8668, -23.092) centre (-3.816, -23.092) ccw
  arc A5621 (-3.8668, -24.108) -> (-3.7652, -24.108) centre (-3.816, -24.108) ccw
  line L2637 (-3.816, -23.092) -> (-1.784, -23.092)
  arc A5622 (-1.784, -23.1428) -> (-1.784, -23.0412) centre (-1.784, -23.092) ccw
  arc A5623 (-3.816, -23.0412) -> (-3.816, -23.1428) centre (-3.816, -23.092) ccw
  line L2638 (-1.784, -23.092) -> (-1.784, -24.108)
  arc A5624 (-1.8348, -24.108) -> (-1.7332, -24.108) centre (-1.784, -24.108) ccw
  arc A5625 (-1.7332, -23.092) -> (-1.8348, -23.092) centre (-1.784, -23.092) ccw
  line L2639 (-7.216, -20.092) -> (-5.184, -20.092)
  arc A5626 (-5.184, -20.1428) -> (-5.184, -20.0412) centre (-5.184, -20.092) ccw
  arc A5627 (-7.216, -20.0412) -> (-7.216, -20.1428) centre (-7.216, -20.092) ccw
  line L2640 (-5.184, -20.092) -> (-5.184, -21.108)
  arc A5628 (-5.2348, -21.108) -> (-5.1332, -21.108) centre (-5.184, -21.108) ccw
  arc A5629 (-5.1332, -20.092) -> (-5.2348, -20.092) centre (-5.184, -20.092) ccw
  line L2641 (-5.184, -21.108) -> (-7.216, -21.108)
  arc A5630 (-7.216, -21.0572) -> (-7.216, -21.1588) centre (-7.216, -21.108) ccw
  arc A5631 (-5.184, -21.1588) -> (-5.184, -21.0572) centre (-5.184, -21.108) ccw
  line L2642 (-7.216, -21.108) -> (-7.216, -20.092)
  arc A5632 (-7.1652, -20.092) -> (-7.2668, -20.092) centre (-7.216, -20.092) ccw
  arc A5633 (-7.2668, -21.108) -> (-7.1652, -21.108) centre (-7.216, -21.108) ccw
  line L2643 (-1.784, -23.108) -> (-3.816, -23.108)
  arc A5634 (-3.816, -23.0572) -> (-3.816, -23.1588) centre (-3.816, -23.108) ccw
  arc A5635 (-1.784, -23.1588) -> (-1.784, -23.0572) centre (-1.784, -23.108) ccw
  line L2644 (-3.816, -23.108) -> (-3.816, -22.092)
  arc A5636 (-3.7652, -22.092) -> (-3.8668, -22.092) centre (-3.816, -22.092) ccw
  arc A5637 (-3.8668, -23.108) -> (-3.7652, -23.108) centre (-3.816, -23.108) ccw
  line L2645 (-3.816, -22.092) -> (-1.784, -22.092)
  arc A5638 (-1.784, -22.1428) -> (-1.784, -22.0412) centre (-1.784, -22.092) ccw
  arc A5639 (-3.816, -22.0412) -> (-3.816, -22.1428) centre (-3.816, -22.092) ccw
  line L2646 (-1.784, -22.092) -> (-1.784, -23.108)
  arc A5640 (-1.8348, -23.108) -> (-1.7332, -23.108) centre (-1.784, -23.108) ccw
  arc A5641 (-1.7332, -22.092) -> (-1.8348, -22.092) centre (-1.784, -22.092) ccw
  line L2647 (-37.316, -50.692) -> (-35.284, -50.692)
  arc A5642 (-35.284, -50.7428) -> (-35.284, -50.6412) centre (-35.284, -50.692) ccw
  arc A5643 (-37.316, -50.6412) -> (-37.316, -50.7428) centre (-37.316, -50.692) ccw
  line L2648 (-35.284, -50.692) -> (-35.284, -51.708)
  arc A5644 (-35.3348, -51.708) -> (-35.2332, -51.708) centre (-35.284, -51.708) ccw
  arc A5645 (-35.2332, -50.692) -> (-35.3348, -50.692) centre (-35.284, -50.692) ccw
  line L2649 (-35.284, -51.708) -> (-37.316, -51.708)
  arc A5646 (-37.316, -51.6572) -> (-37.316, -51.7588) centre (-37.316, -51.708) ccw
  arc A5647 (-35.284, -51.7588) -> (-35.284, -51.6572) centre (-35.284, -51.708) ccw
  line L2650 (-37.316, -51.708) -> (-37.316, -50.692)
  arc A5648 (-37.2652, -50.692) -> (-37.3668, -50.692) centre (-37.316, -50.692) ccw
  arc A5649 (-37.3668, -51.708) -> (-37.2652, -51.708) centre (-37.316, -51.708) ccw
  line L2651 (-37.316, -49.692) -> (-35.284, -49.692)
  arc A5650 (-35.284, -49.7428) -> (-35.284, -49.6412) centre (-35.284, -49.692) ccw
  arc A5651 (-37.316, -49.6412) -> (-37.316, -49.7428) centre (-37.316, -49.692) ccw
  line L2652 (-35.284, -49.692) -> (-35.284, -50.708)
  arc A5652 (-35.3348, -50.708) -> (-35.2332, -50.708) centre (-35.284, -50.708) ccw
  arc A5653 (-35.2332, -49.692) -> (-35.3348, -49.692) centre (-35.284, -49.692) ccw
  line L2653 (-35.284, -50.708) -> (-37.316, -50.708)
  arc A5654 (-37.316, -50.6572) -> (-37.316, -50.7588) centre (-37.316, -50.708) ccw
  arc A5655 (-35.284, -50.7588) -> (-35.284, -50.6572) centre (-35.284, -50.708) ccw
  line L2654 (-37.316, -50.708) -> (-37.316, -49.692)
  arc A5656 (-37.2652, -49.692) -> (-37.3668, -49.692) centre (-37.316, -49.692) ccw
  arc A5657 (-37.3668, -50.708) -> (-37.2652, -50.708) centre (-37.316, -50.708) ccw
  line L2655 (-37.316, -48.692) -> (-35.284, -48.692)
  arc A5658 (-35.284, -48.7428) -> (-35.284, -48.6412) centre (-35.284, -48.692) ccw
  arc A5659 (-37.316, -48.6412) -> (-37.316, -48.7428) centre (-37.316, -48.692) ccw
  line L2656 (-35.284, -48.692) -> (-35.284, -49.708)
  arc A5660 (-35.3348, -49.708) -> (-35.2332, -49.708) centre (-35.284, -49.708) ccw
  arc A5661 (-35.2332, -48.692) -> (-35.3348, -48.692) centre (-35.284, -48.692) ccw
  line L2657 (-35.284, -49.708) -> (-37.316, -49.708)
  arc A5662 (-37.316, -49.6572) -> (-37.316, -49.7588) centre (-37.316, -49.708) ccw
  arc A5663 (-35.284, -49.7588) -> (-35.284, -49.6572) centre (-35.284, -49.708) ccw
  line L2658 (-37.316, -49.708) -> (-37.316, -48.692)
  arc A5664 (-37.2652, -48.692) -> (-37.3668, -48.692) centre (-37.316, -48.692) ccw
  arc A5665 (-37.3668, -49.708) -> (-37.2652, -49.708) centre (-37.316, -49.708) ccw
  line L2659 (-37.316, -47.692) -> (-35.284, -47.692)
  arc A5666 (-35.284, -47.7428) -> (-35.284, -47.6412) centre (-35.284, -47.692) ccw
  arc A5667 (-37.316, -47.6412) -> (-37.316, -47.7428) centre (-37.316, -47.692) ccw
  line L2660 (-35.284, -47.692) -> (-35.284, -48.708)
  arc A5668 (-35.3348, -48.708) -> (-35.2332, -48.708) centre (-35.284, -48.708) ccw
  arc A5669 (-35.2332, -47.692) -> (-35.3348, -47.692) centre (-35.284, -47.692) ccw
  line L2661 (-35.284, -48.708) -> (-37.316, -48.708)
  arc A5670 (-37.316, -48.6572) -> (-37.316, -48.7588) centre (-37.316, -48.708) ccw
  arc A5671 (-35.284, -48.7588) -> (-35.284, -48.6572) centre (-35.284, -48.708) ccw
  line L2662 (-37.316, -48.708) -> (-37.316, -47.692)
  arc A5672 (-37.2652, -47.692) -> (-37.3668, -47.692) centre (-37.316, -47.692) ccw
  arc A5673 (-37.3668, -48.708) -> (-37.2652, -48.708) centre (-37.316, -48.708) ccw
  line L2663 (-37.316, -46.692) -> (-35.284, -46.692)
  arc A5674 (-35.284, -46.7428) -> (-35.284, -46.6412) centre (-35.284, -46.692) ccw
  arc A5675 (-37.316, -46.6412) -> (-37.316, -46.7428) centre (-37.316, -46.692) ccw
  line L2664 (-35.284, -46.692) -> (-35.284, -47.708)
  arc A5676 (-35.3348, -47.708) -> (-35.2332, -47.708) centre (-35.284, -47.708) ccw
  arc A5677 (-35.2332, -46.692) -> (-35.3348, -46.692) centre (-35.284, -46.692) ccw
  line L2665 (-35.284, -47.708) -> (-37.316, -47.708)
  arc A5678 (-37.316, -47.6572) -> (-37.316, -47.7588) centre (-37.316, -47.708) ccw
  arc A5679 (-35.284, -47.7588) -> (-35.284, -47.6572) centre (-35.284, -47.708) ccw
  line L2666 (-37.316, -47.708) -> (-37.316, -46.692)
  arc A5680 (-37.2652, -46.692) -> (-37.3668, -46.692) centre (-37.316, -46.692) ccw
  arc A5681 (-37.3668, -47.708) -> (-37.2652, -47.708) centre (-37.316, -47.708) ccw
  line L2667 (-37.316, -45.692) -> (-35.284, -45.692)
  arc A5682 (-35.284, -45.7428) -> (-35.284, -45.6412) centre (-35.284, -45.692) ccw
  arc A5683 (-37.316, -45.6412) -> (-37.316, -45.7428) centre (-37.316, -45.692) ccw
  line L2668 (-35.284, -45.692) -> (-35.284, -46.708)
  arc A5684 (-35.3348, -46.708) -> (-35.2332, -46.708) centre (-35.284, -46.708) ccw
  arc A5685 (-35.2332, -45.692) -> (-35.3348, -45.692) centre (-35.284, -45.692) ccw
  line L2669 (-35.284, -46.708) -> (-37.316, -46.708)
  arc A5686 (-37.316, -46.6572) -> (-37.316, -46.7588) centre (-37.316, -46.708) ccw
  arc A5687 (-35.284, -46.7588) -> (-35.284, -46.6572) centre (-35.284, -46.708) ccw
  line L2670 (-37.316, -46.708) -> (-37.316, -45.692)
  arc A5688 (-37.2652, -45.692) -> (-37.3668, -45.692) centre (-37.316, -45.692) ccw
  arc A5689 (-37.3668, -46.708) -> (-37.2652, -46.708) centre (-37.316, -46.708) ccw
  line L2671 (-37.316, -44.692) -> (-35.284, -44.692)
  arc A5690 (-35.284, -44.7428) -> (-35.284, -44.6412) centre (-35.284, -44.692) ccw
  arc A5691 (-37.316, -44.6412) -> (-37.316, -44.7428) centre (-37.316, -44.692) ccw
  line L2672 (-35.284, -44.692) -> (-35.284, -45.708)
  arc A5692 (-35.3348, -45.708) -> (-35.2332, -45.708) centre (-35.284, -45.708) ccw
  arc A5693 (-35.2332, -44.692) -> (-35.3348, -44.692) centre (-35.284, -44.692) ccw
  line L2673 (-35.284, -45.708) -> (-37.316, -45.708)
  arc A5694 (-37.316, -45.6572) -> (-37.316, -45.7588) centre (-37.316, -45.708) ccw
  arc A5695 (-35.284, -45.7588) -> (-35.284, -45.6572) centre (-35.284, -45.708) ccw
  line L2674 (-37.316, -45.708) -> (-37.316, -44.692)
  arc A5696 (-37.2652, -44.692) -> (-37.3668, -44.692) centre (-37.316, -44.692) ccw
  arc A5697 (-37.3668, -45.708) -> (-37.2652, -45.708) centre (-37.316, -45.708) ccw
  line L2675 (-37.316, -43.692) -> (-35.284, -43.692)
  arc A5698 (-35.284, -43.7428) -> (-35.284, -43.6412) centre (-35.284, -43.692) ccw
  arc A5699 (-37.316, -43.6412) -> (-37.316, -43.7428) centre (-37.316, -43.692) ccw
  line L2676 (-35.284, -43.692) -> (-35.284, -44.708)
  arc A5700 (-35.3348, -44.708) -> (-35.2332, -44.708) centre (-35.284, -44.708) ccw
  arc A5701 (-35.2332, -43.692) -> (-35.3348, -43.692) centre (-35.284, -43.692) ccw
  line L2677 (-35.284, -44.708) -> (-37.316, -44.708)
  arc A5702 (-37.316, -44.6572) -> (-37.316, -44.7588) centre (-37.316, -44.708) ccw
  arc A5703 (-35.284, -44.7588) -> (-35.284, -44.6572) centre (-35.284, -44.708) ccw
  line L2678 (-37.316, -44.708) -> (-37.316, -43.692)
  arc A5704 (-37.2652, -43.692) -> (-37.3668, -43.692) centre (-37.316, -43.692) ccw
  arc A5705 (-37.3668, -44.708) -> (-37.2652, -44.708) centre (-37.316, -44.708) ccw
  line L2679 (-19.116, 49.008) -> (-17.084, 49.008)
  arc A5706 (-17.084, 48.9572) -> (-17.084, 49.0588) centre (-17.084, 49.008) ccw
  arc A5707 (-19.116, 49.0588) -> (-19.116, 48.9572) centre (-19.116, 49.008) ccw
  line L2680 (-17.084, 49.008) -> (-17.084, 47.992)
  arc A5708 (-17.1348, 47.992) -> (-17.0332, 47.992) centre (-17.084, 47.992) ccw
  arc A5709 (-17.0332, 49.008) -> (-17.1348, 49.008) centre (-17.084, 49.008) ccw
  line L2681 (-17.084, 47.992) -> (-19.116, 47.992)
  arc A5710 (-19.116, 48.0428) -> (-19.116, 47.9412) centre (-19.116, 47.992) ccw
  arc A5711 (-17.084, 47.9412) -> (-17.084, 48.0428) centre (-17.084, 47.992) ccw
  line L2682 (-19.116, 47.992) -> (-19.116, 49.008)
  arc A5712 (-19.0652, 49.008) -> (-19.1668, 49.008) centre (-19.116, 49.008) ccw
  arc A5713 (-19.1668, 47.992) -> (-19.0652, 47.992) centre (-19.116, 47.992) ccw
  line L2683 (-19.116, 50.008) -> (-17.084, 50.008)
  arc A5714 (-17.084, 49.9572) -> (-17.084, 50.0588) centre (-17.084, 50.008) ccw
  arc A5715 (-19.116, 50.0588) -> (-19.116, 49.9572) centre (-19.116, 50.008) ccw
  line L2684 (-17.084, 50.008) -> (-17.084, 48.992)
  arc A5716 (-17.1348, 48.992) -> (-17.0332, 48.992) centre (-17.084, 48.992) ccw
  arc A5717 (-17.0332, 50.008) -> (-17.1348, 50.008) centre (-17.084, 50.008) ccw
  line L2685 (-17.084, 48.992) -> (-19.116, 48.992)
  arc A5718 (-19.116, 49.0428) -> (-19.116, 48.9412) centre (-19.116, 48.992) ccw
  arc A5719 (-17.084, 48.9412) -> (-17.084, 49.0428) centre (-17.084, 48.992) ccw
  line L2686 (-19.116, 48.992) -> (-19.116, 50.008)
  arc A5720 (-19.0652, 50.008) -> (-19.1668, 50.008) centre (-19.116, 50.008) ccw
  arc A5721 (-19.1668, 48.992) -> (-19.0652, 48.992) centre (-19.116, 48.992) ccw
  line L2687 (-24.292, 38.716) -> (-24.292, 36.684)
  arc A5722 (-24.3428, 36.684) -> (-24.2412, 36.684) centre (-24.292, 36.684) ccw
  arc A5723 (-24.2412, 38.716) -> (-24.3428, 38.716) centre (-24.292, 38.716) ccw
  line L2688 (-24.292, 36.684) -> (-25.308, 36.684)
  arc A5724 (-25.308, 36.7348) -> (-25.308, 36.6332) centre (-25.308, 36.684) ccw
  arc A5725 (-24.292, 36.6332) -> (-24.292, 36.7348) centre (-24.292, 36.684) ccw
  line L2689 (-25.308, 36.684) -> (-25.308, 38.716)
  arc A5726 (-25.2572, 38.716) -> (-25.3588, 38.716) centre (-25.308, 38.716) ccw
  arc A5727 (-25.3588, 36.684) -> (-25.2572, 36.684) centre (-25.308, 36.684) ccw
  line L2690 (-25.308, 38.716) -> (-24.292, 38.716)
  arc A5728 (-24.292, 38.6652) -> (-24.292, 38.7668) centre (-24.292, 38.716) ccw
  arc A5729 (-25.308, 38.7668) -> (-25.308, 38.6652) centre (-25.308, 38.716) ccw
  line L2691 (-26.016, 49.108) -> (-23.984, 49.108)
  arc A5730 (-23.984, 49.0572) -> (-23.984, 49.1588) centre (-23.984, 49.108) ccw
  arc A5731 (-26.016, 49.1588) -> (-26.016, 49.0572) centre (-26.016, 49.108) ccw
  line L2692 (-23.984, 49.108) -> (-23.984, 48.092)
  arc A5732 (-24.0348, 48.092) -> (-23.9332, 48.092) centre (-23.984, 48.092) ccw
  arc A5733 (-23.9332, 49.108) -> (-24.0348, 49.108) centre (-23.984, 49.108) ccw
  line L2693 (-23.984, 48.092) -> (-26.016, 48.092)
  arc A5734 (-26.016, 48.1428) -> (-26.016, 48.0412) centre (-26.016, 48.092) ccw
  arc A5735 (-23.984, 48.0412) -> (-23.984, 48.1428) centre (-23.984, 48.092) ccw
  line L2694 (-26.016, 48.092) -> (-26.016, 49.108)
  arc A5736 (-25.9652, 49.108) -> (-26.0668, 49.108) centre (-26.016, 49.108) ccw
  arc A5737 (-26.0668, 48.092) -> (-25.9652, 48.092) centre (-26.016, 48.092) ccw
  arc A5738 (-46.9186, -40.1645) -> (-47.4815, -39.8395) centre (-47.2, -40.002) ccw
  arc A5739 (-47.4815, -39.8395) -> (-46.9186, -40.1645) centre (-47.2, -40.002) ccw
  arc A5740 (-46.9186, -40.1645) -> (-47.4815, -39.8395) centre (-47.2, -40.002) ccw
  arc A5741 (-47.4815, -39.8395) -> (-46.9186, -40.1645) centre (-47.2, -40.002) ccw
  arc A5742 (-45.1676, -40.5795) -> (-45.7305, -40.2545) centre (-45.449, -40.417) ccw
  arc A5743 (-45.7305, -40.2545) -> (-45.1676, -40.5795) centre (-45.449, -40.417) ccw
  arc A5744 (-45.1676, -40.5795) -> (-45.7305, -40.2545) centre (-45.449, -40.417) ccw
  arc A5745 (-45.7305, -40.2545) -> (-45.1676, -40.5795) centre (-45.449, -40.417) ccw
  arc A5746 (-43.5596, -41.3875) -> (-44.1225, -41.0625) centre (-43.841, -41.225) ccw
  arc A5747 (-44.1225, -41.0625) -> (-43.5596, -41.3875) centre (-43.841, -41.225) ccw
  arc A5748 (-43.5596, -41.3875) -> (-44.1225, -41.0625) centre (-43.841, -41.225) ccw
  arc A5749 (-44.1225, -41.0625) -> (-43.5596, -41.3875) centre (-43.841, -41.225) ccw
  arc A5750 (-42.1816, -42.5445) -> (-42.7445, -42.2195) centre (-42.463, -42.382) ccw
  arc A5751 (-42.7445, -42.2195) -> (-42.1816, -42.5445) centre (-42.463, -42.382) ccw
  arc A5752 (-42.1816, -42.5445) -> (-42.7445, -42.2195) centre (-42.463, -42.382) ccw
  arc A5753 (-42.7445, -42.2195) -> (-42.1816, -42.5445) centre (-42.463, -42.382) ccw
  arc A5754 (-41.1066, -43.9875) -> (-41.6695, -43.6625) centre (-41.388, -43.825) ccw
  arc A5755 (-41.6695, -43.6625) -> (-41.1066, -43.9875) centre (-41.388, -43.825) ccw
  arc A5756 (-41.1066, -43.9875) -> (-41.6695, -43.6625) centre (-41.388, -43.825) ccw
  arc A5757 (-41.6695, -43.6625) -> (-41.1066, -43.9875) centre (-41.388, -43.825) ccw
  arc A5758 (-40.3946, -45.6395) -> (-40.9575, -45.3145) centre (-40.676, -45.477) ccw
  arc A5759 (-40.9575, -45.3145) -> (-40.3946, -45.6395) centre (-40.676, -45.477) ccw
  arc A5760 (-40.3946, -45.6395) -> (-40.9575, -45.3145) centre (-40.676, -45.477) ccw
  arc A5761 (-40.9575, -45.3145) -> (-40.3946, -45.6395) centre (-40.676, -45.477) ccw
  arc A5762 (-40.0816, -47.4115) -> (-40.6445, -47.0865) centre (-40.363, -47.249) ccw
  arc A5763 (-40.6445, -47.0865) -> (-40.0816, -47.4115) centre (-40.363, -47.249) ccw
  arc A5764 (-40.0816, -47.4115) -> (-40.6445, -47.0865) centre (-40.363, -47.249) ccw
  arc A5765 (-40.6445, -47.0865) -> (-40.0816, -47.4115) centre (-40.363, -47.249) ccw
  arc A5766 (-40.1866, -49.2085) -> (-40.7495, -48.8835) centre (-40.468, -49.046) ccw
  arc A5767 (-40.7495, -48.8835) -> (-40.1866, -49.2085) centre (-40.468, -49.046) ccw
  arc A5768 (-40.1866, -49.2085) -> (-40.7495, -48.8835) centre (-40.468, -49.046) ccw
  arc A5769 (-40.7495, -48.8835) -> (-40.1866, -49.2085) centre (-40.468, -49.046) ccw
  arc A5770 (-40.7026, -50.9325) -> (-41.2655, -50.6075) centre (-40.984, -50.77) ccw
  arc A5771 (-41.2655, -50.6075) -> (-40.7026, -50.9325) centre (-40.984, -50.77) ccw
  arc A5772 (-40.7026, -50.9325) -> (-41.2655, -50.6075) centre (-40.984, -50.77) ccw
  arc A5773 (-41.2655, -50.6075) -> (-40.7026, -50.9325) centre (-40.984, -50.77) ccw
  arc A5774 (-41.6026, -52.4905) -> (-42.1655, -52.1655) centre (-41.884, -52.328) ccw
  arc A5775 (-42.1655, -52.1655) -> (-41.6026, -52.4905) centre (-41.884, -52.328) ccw
  arc A5776 (-41.6026, -52.4905) -> (-42.1655, -52.1655) centre (-41.884, -52.328) ccw
  arc A5777 (-42.1655, -52.1655) -> (-41.6026, -52.4905) centre (-41.884, -52.328) ccw
  arc A5778 (-42.8366, -53.7995) -> (-43.3995, -53.4745) centre (-43.118, -53.637) ccw
  arc A5779 (-43.3995, -53.4745) -> (-42.8366, -53.7995) centre (-43.118, -53.637) ccw
  arc A5780 (-42.8366, -53.7995) -> (-43.3995, -53.4745) centre (-43.118, -53.637) ccw
  arc A5781 (-43.3995, -53.4745) -> (-42.8366, -53.7995) centre (-43.118, -53.637) ccw
  arc A5782 (-44.3406, -54.7885) -> (-44.9035, -54.4635) centre (-44.622, -54.626) ccw
  arc A5783 (-44.9035, -54.4635) -> (-44.3406, -54.7885) centre (-44.622, -54.626) ccw
  arc A5784 (-44.3406, -54.7885) -> (-44.9035, -54.4635) centre (-44.622, -54.626) ccw
  arc A5785 (-44.9035, -54.4635) -> (-44.3406, -54.7885) centre (-44.622, -54.626) ccw
  arc A5786 (-46.0316, -55.4035) -> (-46.5945, -55.0785) centre (-46.313, -55.241) ccw
  arc A5787 (-46.5945, -55.0785) -> (-46.0316, -55.4035) centre (-46.313, -55.241) ccw
  arc A5788 (-46.0316, -55.4035) -> (-46.5945, -55.0785) centre (-46.313, -55.241) ccw
  arc A5789 (-46.5945, -55.0785) -> (-46.0316, -55.4035) centre (-46.313, -55.241) ccw
  arc A5790 (-47.8186, -55.6125) -> (-48.3815, -55.2875) centre (-48.1, -55.45) ccw